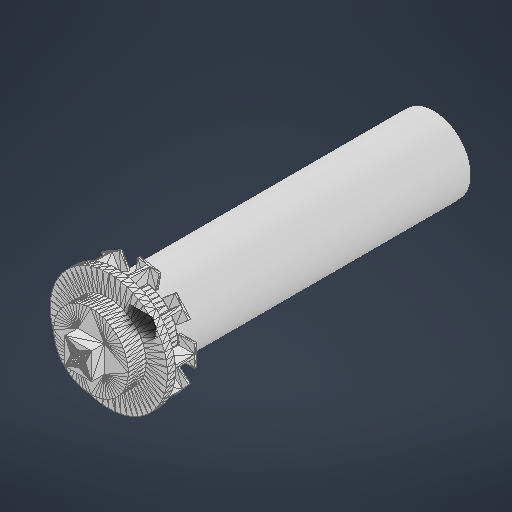
# Autodesk Inventor part: Rodamiento_Motor_X2
Saved by Autodesk Inventor 2026.1 (Build 301233020, 233B)
## iProperties
Created: 2025-11-18
Part Number: Rodamiento_Motor_X2
Material: Genérico
Document SubType Name: Modeling
Designer: Asus
Density: 1 g/cm^3
Appearance: Valor por defecto
Author: Asus
Autodesk Inventor part; units mm, degrees
ref_plane "YZ Plane" through (0, 0, 0) normal (1, 0, 0) x (0, 1, 0)
ref_plane "XZ Plane" through (0, 0, 0) normal (0, 1, 0) x (-1, 0, 0)
ref_plane "XY Plane" through (0, 0, 0) normal (0, 0, 1) x (1, 0, 0)
sketch "Boceto1" plane through (2.1662, 2, 0) normal (0, 0, -1) x (-1, 0, 0)
  line L0 (4.3355, -4) -> (-0.0031, -4)
  line L1 (4.3355, 0) -> (-0.0031, 0)
  arc A0 (4.3355, -4) -> (4.3355, 0) centre (2.1662, -2) ccw
  arc A1 (-0.0031, 0) -> (-0.0031, -4) centre (2.1662, -2) ccw
  circle A2 centre (2.1662, -2) radius 6.9999
  constraints: 4 end point, 4 point on circle, 3 centre point, 2 coincident, 1 horizontal, 1 parallel
extrude "Extrusión1" add sketch "Boceto1" along normal blind 55
